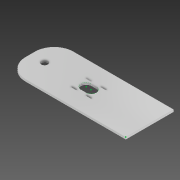
# Autodesk Inventor part: bovenarm - links
Saved by Autodesk Inventor 2020 (Build 240168000, 168)
## iProperties
Created: 2020-05-18
Part Number: bovenarm - links
Material: Generic
Document SubType Name: Modeling
Designer: stefa
Density: 1 g/cm^3
Appearance: Aluminum - Polished
Author: stefa
Autodesk Inventor part; units mm, degrees
ref_plane "YZ Plane" through (0, 0, 0) normal (1, 0, 0) x (0, 1, 0)
ref_plane "XZ Plane" through (0, 0, 0) normal (0, 1, 0) x (-1, 0, 0)
ref_plane "XY Plane" through (0, 0, 0) normal (0, 0, 1) x (1, 0, 0)
sketch "Sketch1" plane through (0, 0, 0) normal (0, 1, 0) x (-1, 0, 0)
  line L0 (0, 0) -> (250, 0)
  line L1 (250, 0) -> (250, -100)
  line L2 (250, -100) -> (0, -100)
  line L3 (0, -100) -> (0, 0)
  circle A0 centre (220, -50) radius 7
  line L4 (132.636, -50) -> (122.636, -50) construction
  line L5 (132.636, -38.9) -> (122.636, -38.9)
  line L6 (122.636, -61.1) -> (132.636, -61.1)
  arc A1 (132.636, -61.1) -> (132.636, -38.9) centre (132.636, -50) ccw
  arc A2 (122.636, -38.9) -> (122.636, -61.1) centre (122.636, -50) ccw
  line L7 (148.136, -65.5) -> (138.136, -65.5) construction
  line L8 (148.136, -64.2) -> (138.136, -64.2)
  line L9 (138.136, -66.8) -> (148.136, -66.8)
  arc A3 (148.136, -66.8) -> (148.136, -64.2) centre (148.136, -65.5) ccw
  arc A4 (138.136, -64.2) -> (138.136, -66.8) centre (138.136, -65.5) ccw
  line L10 (107.136, -66.8) -> (117.136, -66.8)
  arc A5 (117.136, -66.8) -> (117.136, -64.2) centre (117.136, -65.5) ccw
  line L11 (117.136, -65.5) -> (107.136, -65.5) construction
  line L12 (117.136, -64.2) -> (107.136, -64.2)
  arc A6 (107.136, -64.2) -> (107.136, -66.8) centre (107.136, -65.5) ccw
  line L13 (138.136, -35.8) -> (148.136, -35.8)
  arc A7 (148.136, -35.8) -> (148.136, -33.2) centre (148.136, -34.5) ccw
  line L14 (148.136, -34.5) -> (138.136, -34.5) construction
  line L15 (148.136, -33.2) -> (138.136, -33.2)
  arc A8 (138.136, -33.2) -> (138.136, -35.8) centre (138.136, -34.5) ccw
  line L16 (107.136, -35.8) -> (117.136, -35.8)
  arc A9 (117.136, -35.8) -> (117.136, -33.2) centre (117.136, -34.5) ccw
  line L17 (117.136, -34.5) -> (107.136, -34.5) construction
  line L18 (117.136, -33.2) -> (107.136, -33.2)
  arc A10 (107.136, -33.2) -> (107.136, -35.8) centre (107.136, -34.5) ccw
  point P0 (127.636, -50)
  point P1 (143.136, -65.5)
  point P2 (112.136, -65.5)
  point P3 (143.136, -34.5)
  point P4 (112.136, -34.5)
  dimension "d0" = 250
  dimension "d1" = 100
  dimension "d16" = 14
  dimension "d18" = 50
  dimension "d24" = 22.2
  dimension "d25" = 2.6
  dimension "d26" = 10
  dimension "d27" = 10
  dimension "d28" = 92.364
  dimension "d29" = 50
  dimension "d30" = 30
  dimension "d31" = 15.5
  dimension "d32" = 15.5
  dimension "d35" = 31
  dimension "d38" = 31
  constraints: 48 end point, 20 point on circle, 11 centre point, 8 tangent, 5 parallel, 3 horizontal, 2 midpoint, 1 perpendicular, 1 vertical, 36 other
  measures "d0" distance of L1.end L2.end
  measures "d1" distance of L0.end L1.end
  measures "d16" diameter of A0
  measures "d18" distance from line of L0 A0.centre
  measures "d24" diameter of A2
  measures "d25" diameter of A4
  measures "d26" distance of L9.start L9.end
  measures "d27" distance of L6.start L6.end
  measures "d28" distance of A0.centre point (127.636, -50)
  measures "d29" distance from line of L0 point (127.636, -50)
  measures "d30" distance from line of L1 A0.centre
  measures "d31" horizontal distance of point (127.636, -50) point (143.136, -65.5)
  measures "d32" horizontal distance of point (143.136, -65.5) point (127.636, -50)
  measures "d35" distance of L9.start L10.start
  measures "d38" distance of L9.start L13.start
extrude "Extrusion1" add sketch "Sketch1" along normal blind 4
sketch "Sketch3" plane through (0, 4, 0) normal (0, 1, 0) x (1, 0, 0)
  line L0 (-143.736, 50) -> (-111.536, 50) construction
  arc A0 (-132.636, 61.1) -> (-132.636, 38.9) centre (-132.636, 50) ccw construction
  arc A1 (-122.636, 38.9) -> (-122.636, 61.1) centre (-122.636, 50) ccw construction
  point P0 (0, 0)
  constraints: 2 end point, 2 point on circle, 1 horizontal
fillet "Fillet1" radius 40 2 edges at (-250, 2, 0) (-250, 2, -100)
equation "\"d18\" = 0.5 * d1"
body "Solid1"
